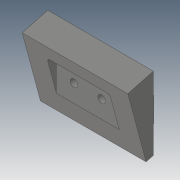
# Autodesk Inventor part: DHC-1500-FF-02-003
Saved by Autodesk Inventor 2018.3 (Build 223284000, 284)
## iProperties
Created: 2018-07-06
Part Number: DHC-1500-FF-02-003
Material: A36
Document SubType Name: Sheet Metal
Designer: R.B.
Stock Number: =<Thickness> - <Material>
Mass: 11271.5 g
Surface Area: 1623.34 cm^2
Volume: 1444 cm^3
Density: 7.80573 g/cm^3
Sheet Metal Rule: Default
Appearance: A36
Thickness: 0.250 in
Author: R.B.
Autodesk Inventor part; units mm, degrees
ref_plane "Right" through (0, 0, 0) normal (1, 0, 0) x (0, 1, 0)
ref_plane "Top" through (0, 0, 0) normal (0, 1, 0) x (-1, 0, 0)
ref_plane "Front" through (0, 0, 0) normal (0, 0, 1) x (1, 0, 0)
sketch "Sketch1" plane through (0, 0, 0) normal (1, 0, 0) x (0, 1, 0)
  line L0 (-40, 15) -> (40, 15)
  line L1 (40, 15) -> (40, -15)
  line L2 (40, -15) -> (-40, -15)
  line L3 (-40, -15) -> (-40, 15)
  line L4 (-40, 15) -> (40, -15) construction
  line L5 (40, 15) -> (-40, -15) construction
  point P0 (0, 0)
  dimension "d0" = 30
  dimension "d1" = 80
  constraints: 12 end point, 2 midpoint, 2 parallel, 1 horizontal, 1 perpendicular
  measures "d0" distance of L0.end L1.end
  measures "d1" distance of L1.end L2.end
extrude "Extrusion1" add sketch "Sketch1" along normal mid plane 140.5
sketch "Sketch2" plane through (-70.25, -40, 15) normal (0, 0, 1) x (1, 0, 0)
  line L0 (140.5, 80) -> (0, 80) construction
  line L1 (0, 0) -> (0, 80) construction
  line L2 (0, 80) -> (0, 58.75)
  line L3 (0, 58.75) -> (34, 80)
  line L4 (34, 80) -> (0, 80)
  line L5 (0, 21.25) -> (0, 0)
  line L6 (0, 0) -> (34, 0)
  line L7 (34, 0) -> (0, 21.25)
  point P0 (70.25, 40)
  dimension "d4" = 37.5
  dimension "d5" = 106.5
  dimension "d6" = 147.995
  constraints: 12 end point, 2 equal length, 2 perpendicular, 2 point on line, 2 vertical
  measures "d4" distance of L5.start L2.end
  measures "d5" distance of L3.end L0.start
  measures "d6" angle of L3 L0
extrude "Extrusion2" cut sketch "Sketch2" against normal through all
sketch "Sketch3" plane through (70.25, -40, 15) normal (0, 0, 1) x (1, 0, 0)
  line L0 (0, 80) -> (0, 0) construction
  line L1 (-140.5, 21.25) -> (-140.5, 58.75) construction
  line L2 (-140.5, 57.1) -> (0, 57.1)
  line L3 (0, 57.1) -> (0, 22.9)
  line L4 (0, 22.9) -> (-140.5, 22.9)
  line L5 (-140.5, 22.9) -> (-140.5, 57.1)
  point P0 (-70.25, 40)
  point P1 (-140.5, 40)
  dimension "d9" = 34.2
  constraints: 8 end point, 2 parallel, 2 point on line, 1 horizontal, 1 horizontal alignment, 1 midpoint, 1 perpendicular
  measures "d9" distance between parallel lines of L4 L2
extrude "Extrusion3" cut sketch "Sketch3" against normal blind 2
sketch "Sketch4" plane through (-36.25, 40, 15) normal (0, 0, 1) x (1, 0, 0)
  line L0 (106.5, -57.1) -> (-34, -57.1) construction
  line L1 (-34, -58.75) -> (-34, -57.1) construction
  line L2 (-34, -58.75) -> (0, -80) construction
  line L3 (0, -80) -> (106.5, -80) construction
  line L4 (106.5, -57.1) -> (106.5, -80) construction
  line L5 (-34, -22.9) -> (106.5, -22.9) construction
  line L6 (-34, -57.1) -> (-34, -22.9) construction
  line L7 (106.5, -57.1) -> (-34, -57.1) construction
  line L8 (106.5, -22.9) -> (106.5, -57.1) construction
  line L9 (106.5, -22) -> (80.5, -22)
  line L10 (80.5, -22) -> (80.5, -58)
  line L11 (80.5, -58) -> (106.5, -58)
  line L12 (106.5, -58) -> (106.5, -22)
  line L13 (85.625, -21.875) -> (85.625, -58.125) construction
  line L14 (90.75, -21.875) -> (90.75, -58.125)
  line L15 (80.5, -58.125) -> (80.5, -21.875)
  arc A0 (90.75, -21.875) -> (80.5, -21.875) centre (85.625, -21.875) ccw
  arc A1 (80.5, -58.125) -> (90.75, -58.125) centre (85.625, -58.125) ccw
  point P0 (36.25, -40)
  point P1 (106.5, -40)
  point P2 (85.625, -40)
  point P3 (80.5, -40)
  dimension "d12" = 36
  dimension "d13" = 26
  dimension "d14" = 46.5
  dimension "d15" = 15.75
  constraints: 16 end point, 5 midpoint, 4 point on circle, 4 tangent, 3 parallel, 2 centre point, 2 perpendicular, 1 horizontal, 1 vertical
  measures "d12" distance of L9.end L10.end
  measures "d13" distance of L10.end L11.end
  measures "d15" distance between parallel lines of L8 L14
extrude "Extrusion4" cut sketch "Sketch4" against normal blind 9.5
sketch "Sketch5" plane through (70.25, -40, 13) normal (0, 0, 1) x (1, 0, 0)
  line L0 (-26, 22.9) -> (-26, 57.1) construction
  line L1 (-15.75, 58) -> (0, 58) construction
  line L2 (-15.75, 58.125) -> (-15.75, 58) construction
  arc A0 (-15.75, 58.125) -> (-26, 58.125) centre (-20.875, 58.125) ccw construction
  line L3 (-26, 21.875) -> (-26, 58.125) construction
  arc A1 (-26, 21.875) -> (-15.75, 21.875) centre (-20.875, 21.875) ccw construction
  line L4 (-15.75, 22) -> (-15.75, 21.875) construction
  line L5 (0, 22) -> (-15.75, 22) construction
  line L6 (0, 58) -> (0, 22) construction
  line L7 (-90.5, 40) -> (-50.5, 40)
  circle A2 centre (-90.5, 40) radius 4.25
  circle A3 centre (-50.5, 40) radius 4.25
  point P0 (-70.25, 40)
  dimension "d18" = 8.5
  dimension "d19" = 48.5
  dimension "d20" = 20.25
  dimension "d23" = 50.5
  dimension "d24" = 40
  constraints: 2 centre point, 2 coincident, 2 end point, 1 equal radius, 1 horizontal, 1 point on line
  measures "d18" diameter of A3
  measures "d20" distance edge to line of A3 L0
  measures "d23" distance from line of A3.centre L6
  measures "d24" distance of L7.start L7.end
hole "Hole1" at (-20.25, 0, 13) at (19.75, 0, 13) direction (0, 0, -1) diameter 8.509 end through all
sketch "Sketch6" plane through (70.25, 0, 0) normal (1, 0, 0) x (0, 0, -1)
  line L0 (15, -40) -> (15, 40) construction
  line L1 (15, 40) -> (-15, 40) construction
  line L2 (15, -40) -> (-6.4359, 40)
  line L3 (-6.4359, 40) -> (15, 40)
  line L4 (15, 40) -> (15, -40)
  point P0 (0, 0)
  dimension "d32" = 15
  constraints: 6 end point, 1 collinear, 1 perpendicular, 1 point on line
  measures "d32" angle of L2 L0
extrude "Extrusion5" cut sketch "Sketch6" against normal through all
sketch "Sketch7" plane through (-36.25, -40, 15) normal (0, 0, 1) x (1, 0, 0)
  line L0 (80.5, 57.1) -> (80.5, 58.125) construction
  arc A0 (90.75, 58.125) -> (80.5, 58.125) centre (85.625, 58.125) ccw construction
  line L1 (90.75, 58.125) -> (90.75, 58) construction
  line L2 (90.75, 58) -> (106.5, 58) construction
  line L3 (106.5, 80) -> (106.5, 58) construction
  line L4 (106.5, 80) -> (0, 80) construction
  line L5 (0, 80) -> (-34, 58.75) construction
  line L6 (-34, 57.1) -> (-34, 58.75) construction
  line L7 (-34, 57.1) -> (80.5, 57.1) construction
  line L8 (106.5, 80) -> (0, 80) construction
  line L9 (106.5, 0) -> (106.5, 80)
  line L10 (106.5, 80) -> (0, 80) construction
  line L11 (106.5, 80) -> (0, 80)
  line L12 (0, 80) -> (-34, 58.75)
  line L13 (0, 80) -> (-34, 58.75) construction
  line L14 (-34, 58.75) -> (-34, 21.25)
  line L15 (-34, 21.25) -> (0, 0)
  line L16 (106.5, 0) -> (106.5, 80) construction
  line L17 (0, 0) -> (106.5, 0)
  point P0 (36.25, 40)
  constraints: 12 end point, 2 horizontal, 1 collinear, 1 perpendicular, 1 vertical
extrude "Extrusion6" add sketch "Sketch7" against normal up to surface (30 mm away) separate body
sketch "Sketch8" plane through (70.25, -40, 13) normal (0, 0, 1) x (1, 0, 0)
  circle A0 centre (-90.5, 40) radius 4.2545 construction
  circle A1 centre (-50.5, 40) radius 4.2545 construction
  line L0 (-26, 22.9) -> (-26, 57.1) construction
  line L1 (-140.5, 57.1) -> (-26, 57.1) construction
  line L2 (-140.5, 22.9) -> (-140.5, 57.1) construction
  line L3 (-26, 22.9) -> (-140.5, 22.9) construction
  line L4 (0, 58) -> (0, 22) construction
  line L5 (12.7, 57.1) -> (-162.725, 57.1)
  line L6 (-162.725, 57.1) -> (-162.725, 22.9)
  line L7 (-162.725, 22.9) -> (12.7, 22.9)
  point P0 (-70.25, 40)
  dimension "d39" = 22.225
  dimension "d40" = 12.7
  constraints: 6 end point, 2 perpendicular, 2 point on line, 1 horizontal, 1 vertical alignment
  measures "d39" distance between parallel lines of L6 L2
  measures "d40" distance from line of L4 L5.start
sketch "Sketch9" plane through (70.25, 40, 6.4359) normal (0, 0.258819, -0.9659258) x (-1, 0, 0)
  line L0 (140.5, -60.8225) -> (106.5, -82.8221) construction
  line L1 (140.5, -21.9996) -> (140.5, -60.8225) construction
  line L2 (106.5, 0) -> (140.5, -21.9996) construction
  line L3 (0, 0) -> (106.5, 0) construction
  line L4 (0, -82.8221) -> (0, 0) construction
  line L5 (0, -82.8221) -> (106.5, -82.8221) construction
  ellipse E0 centre (90.5, -41.411) end of major axis (90.5, -37.0065) minor radius 4.2545 construction
  ellipse E1 centre (50.5, -41.411) end of major axis (50.5, -37.0065) minor radius 4.2545 construction
  line L6 (0, -41.411) -> (140.5, -41.411)
  point P0 (70.25, -40.3028)
  constraints: 2 end point, 2 midpoint, 2 other
sketch "Sketch10" plane through (-36.25, -40, 15) normal (0, 0, 1) x (1, 0, 0)
  line L0 (80.5, 57.1) -> (80.5, 58.125) construction
  arc A0 (90.75, 58.125) -> (80.5, 58.125) centre (85.625, 58.125) ccw construction
  line L1 (90.75, 58.125) -> (90.75, 58) construction
  line L2 (90.75, 58) -> (106.5, 58) construction
  line L3 (106.5, 80) -> (106.5, 58) construction
  line L4 (106.5, 80) -> (0, 80) construction
  line L5 (0, 80) -> (-34, 58.75) construction
  line L6 (-34, 57.1) -> (-34, 58.75) construction
  line L7 (-34, 57.1) -> (80.5, 57.1) construction
  line L8 (90.75, 58) -> (106.5, 58) construction
  line L9 (90.75, 58.125) -> (90.75, 58) construction
  arc A1 (90.75, 58.125) -> (80.5, 58.125) centre (85.625, 58.125) ccw construction
  line L10 (80.5, 21.875) -> (80.5, 58.125) construction
  arc A2 (80.5, 21.875) -> (90.75, 21.875) centre (85.625, 21.875) ccw construction
  line L11 (90.75, 22) -> (90.75, 21.875) construction
  line L12 (106.5, 22) -> (90.75, 22) construction
  line L13 (106.5, 58) -> (106.5, 22) construction
  circle A3 centre (16, 40) radius 4.2545 construction
  circle A4 centre (56, 40) radius 4.2545 construction
  line L14 (80.5, 22.9) -> (80.5, 57.1) construction
  line L15 (-34, 57.1) -> (80.5, 57.1) construction
  line L16 (-34, 22.9) -> (-34, 57.1) construction
  line L17 (80.5, 22.9) -> (-34, 22.9) construction
  line L18 (112.45, 94.0004) -> (-39.95, 94.0004)
  line L19 (-39.95, 94.0004) -> (-39.95, -14.0004)
  line L20 (-39.95, -14.0004) -> (112.45, -14.0004)
  line L21 (112.45, -14.0004) -> (112.45, 94.0004)
  line L22 (-34, 40) -> (106.5, 40) construction
  line L23 (112.45, 94.0004) -> (-39.95, -14.0004) construction
  point P0 (36.25, 40)
  point P1 (36.25, 40)
  dimension "d41" = 152.4
  dimension "d42" = 108.0008
  constraints: 12 end point, 3 midpoint, 2 parallel, 1 coincident, 1 horizontal, 1 perpendicular
  measures "d41" distance of L18.start L18.end
  measures "d42" distance of L20.end L18.start
extrude "Extrusion7" add sketch "Sketch10" along normal blind 36.8046 separate body
sketch "Sketch13" plane through (76.2, -54.0004, 15) normal (1, 0, 0) x (0, 0, -1)
  line L0 (0, 0) -> (0, 108.0008) construction
  line L1 (0, 0) -> (-36.8046, 0) construction
  line L2 (-10.5083, 0) -> (-36.8046, 98.139)
  line L3 (30, 14.0004) -> (8.5641, 94.0004) construction
  line L4 (-36.8046, 108.0008) -> (-36.8046, 0)
  line L5 (-10.5083, 0) -> (-36.8046, 0)
  line L6 (-36.8046, 0) -> (-36.8046, 108.0008) construction
  line L7 (0, 108.0008) -> (-36.8046, 98.139)
  line L8 (0, 108.0008) -> (-36.8046, 108.0008)
  line L9 (-10.5083, 0) -> (0, 2.8157)
  line L10 (0, 2.8157) -> (0, 0)
  line L11 (0, 0) -> (-10.5083, 0)
  line L12 (-36.8046, 98.139) -> (-10.5083, 0)
  line L13 (-10.5083, 0) -> (-36.8046, 0)
  line L14 (-36.8046, 0) -> (-36.8046, 98.139)
  line L15 (0, 108.0008) -> (-36.8046, 108.0008) construction
  line L16 (0, 108.0008) -> (-36.8046, 98.139)
  line L17 (-36.8046, 98.139) -> (-36.8046, 108.0008)
  line L18 (-36.8046, 108.0008) -> (0, 108.0008)
  point P0 (15, 54.0004)
  dimension "d67" = 101.601
  dimension "d75" = 38.1029
  constraints: 28 end point, 6 collinear, 5 perpendicular, 3 point on line, 1 parallel, 1 vertical
  measures "d67" distance of L2.start L2.end
  measures "d75" distance of L0.end L2.end
extrude "Extrusion9" cut sketch "Sketch13" against normal through all bodies 3
ref_plane "Work Plane1" through (-36.25, -40, 33.1737) normal (0, 0, -1) x (-1, 0, 0)
sketch "Sketch12" plane through (-36.25, -40, 51.8046) normal (0, 0, 1) x (1, 0, 0)
  circle A0 centre (16, 40) radius 4.2545 construction
  circle A1 centre (56, 40) radius 4.2545 construction
  line L0 (80.5, 22.9) -> (80.5, 57.1) construction
  line L1 (-34, 57.1) -> (80.5, 57.1) construction
  line L2 (-34, 22.9) -> (-34, 57.1) construction
  line L3 (80.5, 22.9) -> (-34, 22.9) construction
  point P0 (36.25, 40)
hole "Hole2" at (19.75, 0, 51.8046) at (-20.25, 0, 51.8046) direction (0, 0, -1) diameter 10.9982 end through all bodies 3 clearance for "Socket Head Cap Screw" size "M10" standard "Ansi Metric M Profile"
sketch "Sketch15" plane through (-36.25, -40, 33.1737) normal (0, 0, -1) x (-1, 0, 0)
  circle A0 centre (-56, 40) radius 5.4991 construction
  circle A1 centre (-16, 40) radius 5.4991 construction
  line L0 (9.4, 65.4) -> (-81.4, 65.4)
  line L1 (-81.4, 65.4) -> (-81.4, -10.8)
  line L2 (-81.4, -10.8) -> (9.4, -10.8)
  line L3 (9.4, -10.8) -> (9.4, 65.4)
  line L4 (9.4, 65.4) -> (-81.4, -10.8) construction
  line L5 (-81.4, 65.4) -> (9.4, -10.8) construction
  point P0 (-36, 27.3)
  dimension "d76" = 25.4
  dimension "d77" = 25.4
  dimension "d78" = 25.4
  dimension "d79" = 50.8
  constraints: 12 end point, 2 midpoint, 2 parallel, 1 horizontal, 1 perpendicular
  measures "d76" distance from line of A0.centre L0
  measures "d77" distance from line of A0.centre L1
  measures "d78" distance from line of A1.centre L3
  measures "d79" distance from line of A0.centre L2
extrude "Extrusion11" cut sketch "Sketch15" against normal through all bodies 3
fillet "Fillet1" radius 4.7752 2 edges at (-45.65, 25.4, 39.9786) (45.15, 25.4, 39.9786)
sketch "Sketch16" plane through (-36.25, -40, 15) normal (0, 0, -1) x (-1, 0, 0)
  line L0 (-90.75, 58) -> (-106.5, 58) construction
  line L1 (-90.75, 58.125) -> (-90.75, 58) construction
  arc A0 (-80.5, 58.125) -> (-90.75, 58.125) centre (-85.625, 58.125) ccw construction
  line L2 (-80.5, 21.875) -> (-80.5, 58.125) construction
  arc A1 (-90.75, 21.875) -> (-80.5, 21.875) centre (-85.625, 21.875) ccw construction
  line L3 (-90.75, 22) -> (-90.75, 21.875) construction
  line L4 (-106.5, 22) -> (-90.75, 22) construction
  line L5 (-106.5, 58) -> (-106.5, 22) construction
  circle A2 centre (-16, 40) radius 4.2545 construction
  circle A3 centre (-56, 40) radius 4.2545 construction
  line L6 (-80.5, 22.9) -> (-80.5, 57.1) construction
  line L7 (34, 57.1) -> (-80.5, 57.1) construction
  line L8 (34, 22.9) -> (34, 57.1) construction
  line L9 (-80.5, 22.9) -> (34, 22.9) construction
  line L10 (-106.5, 58) -> (-80.5, 58)
  line L11 (-80.5, 58) -> (-80.5, 22)
  line L12 (-80.5, 22) -> (-106.5, 22)
  line L13 (-106.5, 22) -> (-106.5, 58)
  line L14 (34, 57.1) -> (-80.5, 57.1)
  line L15 (-80.5, 57.1) -> (-80.5, 22.9)
  line L16 (-80.5, 22.9) -> (34, 22.9)
  line L17 (34, 22.9) -> (34, 57.1)
  circle A4 centre (-56, 40) radius 5.4991 construction
  circle A5 centre (-16, 40) radius 5.4991 construction
  circle A6 centre (-16, 40) radius 5.4991
  circle A7 centre (-56, 40) radius 5.4991
  point P0 (-36.25, 40)
  constraints: 16 end point, 4 parallel, 2 centre point, 2 coincident, 2 concentric, 2 horizontal, 2 perpendicular, 1 point on line
extrude "Extrusion13" add sketch "Sketch16" along normal blind 6.35 contours L10 L11 L12 L13 bodies 3
extrude "Extrusion14" add sketch "Sketch16" along normal blind 1.27 contours L14 L17 L16 L11 bodies 3
sketch "Sketch17" plane through (76.2, -51.1847, 15) normal (1, 0, 0) x (0, 0, -1)
  line L0 (-10.5083, -2.8157) -> (0, 0) projected
  line L1 (0, 0) -> (0, 105.1851) projected
  line L2 (0, 105.1851) -> (-36.8046, 95.3233) projected
  line L3 (-36.8046, 95.3233) -> (-10.5083, -2.8157) projected
  line L4 (0, 0) -> (26.2963, 7.0461)
  line L5 (26.2963, 7.0461) -> (0, 105.1851)
  point P0 (15, 51.1847)
  constraints: 4 end point, 1 collinear, 1 perpendicular
extrude "Extrusion15" add sketch "Sketch17" against normal up to surface (152.4 mm away) separate body
equation "\"d52\" = Thickness"
equation "\"BendRadius\" = Thickness"
equation "\"BendReliefWidth\" = 0.5 * Thickness"
equation "\"BendReliefDepth\" = 0.5 * Thickness"
equation "\"CornerReliefSize\" = 4 * Thickness"
equation "\"MinimumRemnant\" = 2 * Thickness"
equation "\"TransitionRadius\" = BendRadius"
equation "\"JacobiRadiusSize\" = BendRadius"
equation "\"Thickness\" = 6.35"
body "Solid1"
body "Solid2"
body "Solid3"
body "Solid4"
